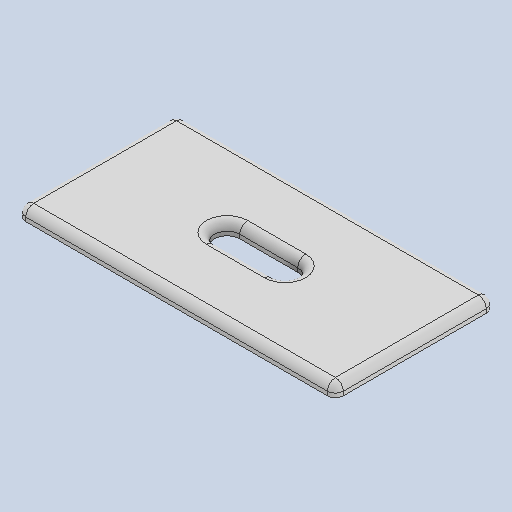
# Autodesk Inventor part: USB-C_Blende
Saved by Autodesk Inventor 2026 (Build 300175000, 175)
## iProperties
Created: 2025-08-28
Part Number: USB-C_Blende
Material: Generisch
Document SubType Name: Modeling
Designer: fabia
Density: 1 g/cm^3
Appearance: Vorgabe
Author: fabia
Autodesk Inventor part; units mm, degrees
ref_plane "YZ Plane" through (0, 0, 0) normal (1, 0, 0) x (0, 1, 0)
ref_plane "XZ Plane" through (0, 0, 0) normal (0, 1, 0) x (-1, 0, 0)
ref_plane "XY Plane" through (0, 0, 0) normal (0, 0, 1) x (1, 0, 0)
sketch "Skizze1" plane through (0, 0, 0) normal (0, 1, 0) x (-1, 0, 0)
  line L0 (3.65, 0) -> (-3.65, 0) construction
  line L1 (3.65, 1.6) -> (-3.65, 1.6)
  line L2 (-3.65, -1.6) -> (3.65, -1.6)
  arc A0 (3.65, -1.6) -> (3.65, 1.6) centre (3.65, 0) ccw
  arc A1 (-3.65, 1.6) -> (-3.65, -1.6) centre (-3.65, 0) ccw
  line L3 (20, -10) -> (-20, -10)
  line L4 (-20, -10) -> (-20, 10)
  line L5 (-20, 10) -> (20, 10)
  line L6 (20, 10) -> (20, -10)
  line L7 (20, -10) -> (-20, 10) construction
  line L8 (-20, -10) -> (20, 10) construction
  point P0 (0, 0)
  point P1 (0, 0)
  point P2 (0, 1.6)
  dimension "d1" = 3.2
  dimension "d2" = 10.5
  dimension "d3" = 40
  dimension "d4" = 20
  constraints: 20 end point, 4 point on circle, 4 tangent, 3 midpoint, 3 parallel, 2 centre point, 2 horizontal, 1 perpendicular, 1 vertical alignment
  measures "d1" diameter of A1
  measures "d3" distance of L4.end L5.end
  measures "d4" distance of L3.end L4.end
extrude "Extrusion1" add sketch "Skizze1" along normal blind 1.5
fillet "Rundung1" radius 1 12 edges at (0, 1.5, 1.6) (-5.25, 1.5, 0) (0, 1.5, -1.6) (5.25, 1.5, 0) (0, 1.5, 10) (-20, 1.5, 0) (-20, 0.75, 10) (0, 1.5, -10) (-20, 0.75, -10) (20, 0.75, 10) (20, 1.5, 0) (20, 0.75, -10)
